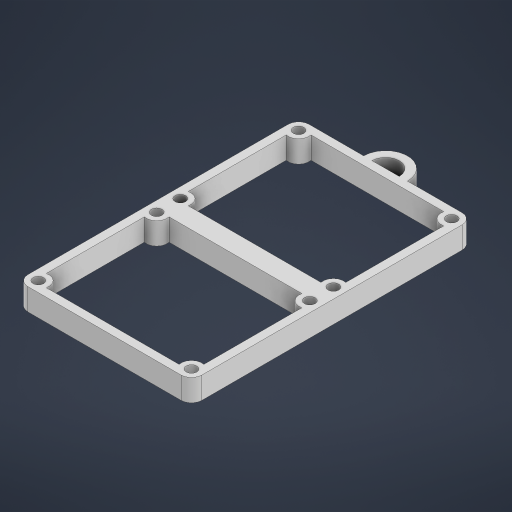
# Autodesk Inventor part: balloonMount_x2
Saved by Autodesk Inventor 2024 (Build 280153000, 153)
## iProperties
Created: 2024-03-19
Part Number: balloonMount_x2
Material: Generic
Document SubType Name: Modeling
Designer: madis
Density: 1 g/cm^3
Appearance: Default
Author: madis
Autodesk Inventor part; units mm, degrees
ref_plane "YZ Plane" through (0, 0, 0) normal (1, 0, 0) x (0, 1, 0)
ref_plane "XZ Plane" through (0, 0, 0) normal (0, 1, 0) x (-1, 0, 0)
ref_plane "XY Plane" through (0, 0, 0) normal (0, 0, 1) x (1, 0, 0)
sketch "Sketch1" plane through (0, 0, 0) normal (0, 1, 0) x (-1, 0, 0)
  circle A0 centre (27.94, -21.59) radius 1.94 construction
  line L0 (3.8945, 0) -> (-7.0745, 0) construction
  line L1 (0, -4.534) -> (0, 5.5912) construction
  circle A1 centre (-27.94, -21.59) radius 1.94 construction
  circle A2 centre (27.94, 21.59) radius 1.94 construction
  circle A3 centre (-27.94, 21.59) radius 1.94 construction
  line L2 (27.94, -25.4) -> (-27.94, -25.4)
  line L3 (31.75, 25.9) -> (-31.75, 25.9) construction
  line L4 (31.75, -21.59) -> (31.75, 25.9)
  line L5 (-31.75, -21.59) -> (-31.75, 25.9)
  line L6 (24.2171, -22.4) -> (-24.2171, -22.4)
  line L7 (24.2171, 22.4) -> (-24.2171, 22.4)
  line L8 (28.75, -17.8671) -> (28.75, 17.8671)
  line L9 (-28.75, -17.8671) -> (-28.75, 17.8671)
  arc A4 (-24.2171, -22.4) -> (-28.75, -17.8671) centre (-27.94, -21.59) ccw
  arc A5 (-31.75, -21.59) -> (-27.94, -25.4) centre (-27.94, -21.59) ccw
  arc A6 (27.94, -25.4) -> (31.75, -21.59) centre (27.94, -21.59) ccw
  arc A7 (28.75, -17.8671) -> (24.2171, -22.4) centre (27.94, -21.59) ccw
  arc A8 (-28.75, 17.8671) -> (-24.2171, 22.4) centre (-27.94, 21.59) ccw
  arc A9 (24.2171, 22.4) -> (28.75, 17.8671) centre (27.94, 21.59) ccw
  circle A10 centre (27.94, 73.39) radius 1.94 construction
  circle A11 centre (-27.94, 73.39) radius 1.94 construction
  circle A12 centre (27.94, 30.21) radius 1.94 construction
  circle A13 centre (-27.94, 30.21) radius 1.94 construction
  line L10 (27.94, 77.2) -> (-27.94, 77.2)
  line L11 (31.75, 73.39) -> (31.75, 25.9)
  line L12 (-31.75, 73.39) -> (-31.75, 25.9)
  line L13 (24.2171, 74.2) -> (-24.2171, 74.2)
  line L14 (24.2171, 29.4) -> (-24.2171, 29.4)
  line L15 (28.75, 69.6671) -> (28.75, 33.9329)
  line L16 (-28.75, 69.6671) -> (-28.75, 33.9329)
  arc A14 (-28.75, 69.6671) -> (-24.2171, 74.2) centre (-27.94, 73.39) ccw
  arc A15 (-27.94, 77.2) -> (-31.75, 73.39) centre (-27.94, 73.39) ccw
  arc A16 (31.75, 73.39) -> (27.94, 77.2) centre (27.94, 73.39) ccw
  arc A17 (24.2171, 74.2) -> (28.75, 69.6671) centre (27.94, 73.39) ccw
  arc A18 (-24.2171, 29.4) -> (-28.75, 33.9329) centre (-27.94, 30.21) ccw
  arc A19 (28.75, 33.9329) -> (24.2171, 29.4) centre (27.94, 30.21) ccw
  arc A20 (-8, -25.4) -> (8, -25.4) centre (0, -25.4) ccw
  arc A21 (-5, -25.4) -> (5, -25.4) centre (0, -25.4) ccw
  point P0 (0, 0)
  dimension "d0" = 3.88
  dimension "d1" = 27.94
  dimension "d2" = 21.59
  dimension "d5" = 55.88
  dimension "d8" = 43.18
  dimension "d11" = 25.4
  dimension "d12" = 31.75
  dimension "d13" = 3
  dimension "d14" = 3
  dimension "d16" = 3.5
  dimension "d17" = 8
  dimension "d18" = 5
  constraints: 34 end point, 28 point on circle, 24 symmetric about line, 22 centre point, 11 coincident, 6 point on line, 5 parallel, 4 horizontal, 4 vertical, 1 concentric, 1 midpoint, 1 tangent, 16 other
  measures "d0" diameter of A0
  measures "d1" horizontal distance of point (0, 0) A0.centre
  measures "d2" vertical distance of point (0, 0) A0.centre
  measures "d5" distance of A0.centre A1.centre
  measures "d8" distance of A0.centre A2.centre
  measures "d11" distance from line of point (0, 0) L2
  measures "d12" distance from line of point (0, 0) L4
  measures "d13" distance between parallel lines of L2 L6
  measures "d14" distance between parallel lines of L4 L8
  measures "d16" distance between parallel lines of L7 L3
  measures "d17" radius of A20
  measures "d18" radius of A21
extrude "Extrusion1" add sketch "Sketch1" along normal blind 8 contours L2 A5 L5 L12 A15 L10 A16 L11 L4 A6 | A20 L2 A21
sketch "Sketch2" plane through (0, 8, 0) normal (0, 1, 0) x (1, 0, 0)
  line L0 (-31.75, 21.59) -> (-31.75, -73.39) projected
  line L1 (-8, 25.4) -> (-27.94, 25.4) projected
  point P0 (0, 0)
  point P1 (-27.94, 21.59)
  dimension "d28" = 3.81
  dimension "d29" = 3.81
  measures "d28" distance from line of L0 point (-27.94, 21.59)
  measures "d29" distance from line of L1 point (-27.94, 21.59)
hole "Hole1" at (-27.94, 8, -21.59) direction (0, -1, 0) diameter 3.88 depth 5.145 tip angle 118
pattern_linear "Rectangular Pattern1" count 2 spacing 55.88 along (1, 0, 0) count 2 spacing 43.18 along (0, 0, 1) of "Hole1"
pattern_linear "Rectangular Pattern2" count 2 spacing 51.8 along (0, 0, 1) of "Hole1", "Rectangular Pattern1"
body "Solid1"
